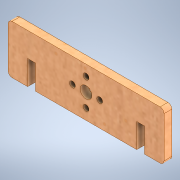
# Autodesk Inventor part: Деталь2
Saved by Autodesk Inventor 2020.1 (Build 241239000, 239)
## iProperties
Created: 2021-08-12
Part Number: Деталь2
Material: Дерево (вишня)
Document SubType Name: Modeling
Designer: Ni3na
Density: 0.63 g/cm^3
Appearance: Вишневое дерево — натуральный — со слабым глянцем
Author: Ni3na
Autodesk Inventor part; units mm, degrees
ref_plane "YZ Plane" through (0, 0, 0) normal (1, 0, 0) x (0, 1, 0)
ref_plane "XZ Plane" through (0, 0, 0) normal (0, 1, 0) x (-1, 0, 0)
ref_plane "XY Plane" through (0, 0, 0) normal (0, 0, 1) x (1, 0, 0)
sketch "Эскиз1" plane through (0, 0, 0) normal (0, 0, 1) x (1, 0, 0)
  line L0 (0, 0) -> (52, 0)
  line L1 (52, 0) -> (52, -25)
  line L2 (52, -25) -> (0, -25)
  line L3 (0, -25) -> (0, 0)
  line L4 (0, -12.5) -> (-4, -12.5)
  line L5 (-4, -12.5) -> (-4, 0)
  line L6 (-4, 0) -> (0, 0)
  line L7 (0, 0) -> (0, -12.5)
  line L8 (-4, 0) -> (-14, 0)
  line L9 (-14, 0) -> (-14, -25)
  line L10 (-14, -25) -> (-4, -25)
  line L11 (-4, -25) -> (-4, 0)
  line L12 (52, -12.5) -> (56, -12.5)
  line L13 (56, -12.5) -> (56, 0)
  line L14 (56, 0) -> (52, 0)
  line L15 (52, 0) -> (52, -12.5)
  line L16 (56, 0) -> (66, 0)
  line L17 (66, 0) -> (66, -25)
  line L18 (66, -25) -> (56, -25)
  line L19 (56, -25) -> (56, 0)
  circle A0 centre (26, -12.5) radius 3
  circle A1 centre (26, -12.5) radius 7
  circle A2 centre (33, -12.5) radius 1.5
  circle A3 centre (19, -12.5) radius 1.5
  circle A4 centre (26, -5.5) radius 1.5
  circle A5 centre (26, -19.5) radius 1.5
  dimension "d0" = 52
  dimension "d1" = 25
  dimension "d2" = 4
  dimension "d3" = 10
  dimension "d4" = 4
  dimension "d5" = 10
  dimension "d9" = 6
  dimension "d10" = 14
  dimension "d11" = 3
  dimension "d12" = 3
  dimension "d13" = 3
  dimension "d14" = 3
  constraints: 40 end point, 10 parallel, 6 centre point, 5 horizontal, 5 perpendicular, 4 point on circle, 2 midpoint, 1 coincident
  measures "d0" distance of L0.start L0.end
  measures "d1" distance of L2.end L0.start
  measures "d2" distance of L5.end L6.end
  measures "d3" distance of L5.end L8.end
  measures "d4" distance of L13.end L14.end
  measures "d5" distance of L13.end L16.end
  measures "d9" diameter of A0
  measures "d10" diameter of A1
  measures "d11" diameter of A2
  measures "d12" diameter of A3
  measures "d13" diameter of A4
  measures "d14" diameter of A5
extrude "Выдавливание1" add sketch "Эскиз1" along normal blind 4 contours L0 L1 L2 L3 | L3 L4 L5 L6 | L14 L13 L12 L1 | L5 L11 L10 L9 L8 | L16 L17 L18 L19 L13 | A2 A1 A5 A3 A4
fillet "Сопряжение1" radius 2 4 edges at (66, 0, 2) (66, -25, 2) (-14, -25, 2) (-14, 0, 2)
